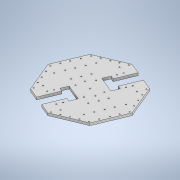
# Autodesk Inventor part: Support bas
Saved by Autodesk Inventor 2020 (Build 240168000, 168)
## iProperties
Created: 2019-11-28
Part Number: Support bas
Material: Générique
Document SubType Name: Modeling
Designer: erwan
Density: 1 g/cm^3
Appearance: Par défaut
Author: erwan
Autodesk Inventor part; units mm, degrees
ref_plane "YZ Plane" through (0, 0, 0) normal (1, 0, 0) x (0, 1, 0)
ref_plane "XZ Plane" through (0, 0, 0) normal (0, 1, 0) x (-1, 0, 0)
ref_plane "XY Plane" through (0, 0, 0) normal (0, 0, 1) x (1, 0, 0)
sketch "Esquisse1" plane through (0, 0, 0) normal (0, 1, 0) x (-1, 0, 0)
  line L0 (174.5381, 0.1913) -> (123.2817, 123.935)
  line L1 (174.5381, 0.1913) -> (123.2817, -123.5523)
  line L2 (123.2817, -123.5523) -> (-0.4619, -174.8087)
  line L3 (-123.2817, -123.935) -> (-174.5381, -0.1913)
  line L4 (-174.5381, -0.1913) -> (-123.2817, 123.5523)
  line L5 (-123.2817, 123.5523) -> (0.4619, 174.8087)
  line L6 (-0.4619, -174.8087) -> (-43.3943, -157.0255)
  line L7 (-123.2817, -123.935) -> (-80.3494, -141.7182)
  line L8 (-1.0786, 88.8554) -> (-12.5591, 61.139)
  line L9 (-12.5591, 61.139) -> (52.1124, 34.3512)
  line L10 (52.1124, 34.3512) -> (63.593, 62.0676)
  line L11 (63.593, 62.0676) -> (49.7348, 67.8078)
  line L12 (49.7348, 67.8078) -> (80.3494, 141.7182)
  line L13 (-1.0786, 88.8554) -> (12.7796, 83.1151)
  line L14 (12.7796, 83.1151) -> (43.3943, 157.0255)
  line L15 (123.2817, 123.935) -> (80.3494, 141.7182)
  line L16 (0.4619, 174.8087) -> (43.3943, 157.0255)
  line L17 (-63.593, -62.0676) -> (-52.1124, -34.3512)
  line L18 (-52.1124, -34.3512) -> (12.5591, -61.139)
  line L19 (12.5591, -61.139) -> (1.0786, -88.8554)
  line L20 (1.0786, -88.8554) -> (-12.7796, -83.1151)
  line L21 (-12.7796, -83.1151) -> (-43.3943, -157.0255)
  line L22 (-63.593, -62.0676) -> (-49.7348, -67.8078)
  line L23 (-49.7348, -67.8078) -> (-80.3494, -141.7182)
  point P0 (0, 0)
  dimension "d113" = 30
  dimension "d114" = 70
  dimension "d115" = 30
  dimension "d116" = 15
  dimension "d117" = 15
  dimension "d120" = 30
  dimension "d121" = 70
  dimension "d122" = 15
  dimension "d123" = 15
  constraints: 48 end point, 8 perpendicular, 2 collinear
  measures "d113" distance of L8.start L8.end
  measures "d114" distance of L8.end L9.end
  measures "d115" distance of L9.end L10.end
  measures "d116" distance of L10.end L11.end
  measures "d117" distance of L8.start L13.end
  measures "d120" distance of L17.start L17.end
  measures "d121" distance of L17.end L18.end
  measures "d122" distance of L19.end L20.end
  measures "d123" distance of L17.start L22.end
extrude "Extrusion1" add sketch "Esquisse1" along normal blind 10
sketch "Esquisse2" plane through (0, 10, 0) normal (0, 1, 0) x (1, 0, 0)
  line L0 (0, 0) -> (135.5137, -56.1316) construction
  line L1 (0, 0) -> (-162.1857, 67.1795) construction
  line L2 (0, 175) -> (-123.7437, -123.7437) construction
  line L3 (0, -175) -> (123.7437, 123.7437) construction
  line L4 (174.5381, 0.1913) -> (-123.2817, 123.5523) construction
  line L5 (-174.5381, -0.1913) -> (123.2817, -123.5523) construction
  line L6 (150.0138, 60.7587) -> (-149.0913, -62.1087) construction
  line L7 (-60.9725, 148.8775) -> (61.8949, -150.2276) construction
  line L8 (-60.9725, 148.8775) -> (-149.0913, -62.1087) construction
  line L9 (61.8949, -150.2276) -> (150.0138, 60.7587) construction
  circle A0 centre (165.8145, -1.0193) radius 2.25
  line L10 (165.8145, -1.0193) -> (116.2638, -120.6454) construction
  circle A1 centre (116.2638, -120.6454) radius 2.25
  circle A2 centre (141.8919, -58.7736) radius 2.25
  circle A3 centre (153.2932, -30.2913) radius 2.25
  circle A4 centre (128.2212, -90.3222) radius 2.25
  line L11 (119.9169, 114.5049) -> (165.8145, -1.0193) construction
  circle A5 centre (119.9169, 114.5049) radius 2.25
  circle A6 centre (142.4969, 57.6709) radius 2.25
  circle A7 centre (130.8905, 86.6335) radius 2.25
  circle A8 centre (153.432, 29.381) radius 2.25
  line L12 (3.8268, -165.7612) -> (116.2638, -120.6454) construction
  circle A9 centre (3.8268, -165.7612) radius 2.25
  circle A10 centre (60.0453, -143.2033) radius 2.25
  circle A11 centre (31.6722, -154.3729) radius 2.25
  circle A12 centre (87.3628, -131.5964) radius 2.25
  line L13 (-164.5381, -0.1913) -> (-114.7462, 120.0168) construction
  circle A13 centre (-164.5381, -0.1913) radius 2.25
  circle A14 centre (-114.7462, 120.0168) radius 2.25
  circle A15 centre (-140.3744, 58.145) radius 2.25
  circle A16 centre (-127.2988, 88.9721) radius 2.25
  circle A17 centre (-152.3708, 28.9413) radius 2.25
  line L14 (-3.8268, 165.7612) -> (-114.7462, 120.0168) construction
  circle A18 centre (-3.8268, 165.7612) radius 2.25
  circle A19 centre (-58.6246, 143.162) radius 2.25
  circle A20 centre (-31.6722, 154.3729) radius 2.25
  circle A21 centre (-87.3628, 131.5964) radius 2.25
  line L15 (-119.9169, -114.5049) -> (-164.5381, -0.1913) construction
  circle A22 centre (-119.9169, -114.5049) radius 2.25
  circle A23 centre (-141.5745, -59.0209) radius 2.25
  circle A24 centre (-130.8905, -86.6335) radius 2.25
  circle A25 centre (-153.432, -29.381) radius 2.25
  circle A26 centre (15.3073, -138.0448) radius 2.25
  circle A27 centre (80.4463, -105.8093) radius 2.25
  circle A28 centre (105.9544, -44.7345) radius 2.25
  circle A29 centre (132.0654, 17.7841) radius 2.25
  circle A30 centre (108.4363, 86.7885) radius 2.25
  circle A31 centre (61.8718, -25.6282) radius 2.25
  circle A32 centre (0, 0) radius 2.25
  circle A33 centre (-15.3073, 138.0448) radius 2.25
  circle A34 centre (-79.1792, 105.2845) radius 2.25
  circle A35 centre (-105.0319, 43.3844) radius 2.25
  circle A36 centre (-130.7983, -18.309) radius 2.25
  circle A37 centre (-61.8718, 25.6282) radius 2.25
  line L16 (183.0548, 10.7676) -> (-121.8254, 137.0531) construction
  line L17 (-121.8254, 137.0531) -> (-183.0548, -10.7676) construction
  line L18 (-183.0548, -10.7676) -> (121.8254, -137.0531) construction
  line L19 (183.0548, 10.7676) -> (121.8254, -137.0531) construction
  line L20 (15.3073, -138.0448) -> (-145.3915, -71.4812) construction
  line L21 (15.3073, -138.0448) -> (52.2625, -153.3522) construction
  circle A38 centre (-108.4363, -86.7885) radius 2.25
  line L22 (-15.6478, 66.748) -> (-57.8915, -35.2375) construction
  line L23 (58.2626, 36.1333) -> (15.8255, -66.3188) construction
  circle A39 centre (37.0441, -15.0928) radius 2.25
  circle A40 centre (-36.7697, 15.7552) radius 2.25
  line L24 (31.2572, -99.5385) -> (49.7348, -107.1922) construction
  line L25 (49.7348, -107.1922) -> (42.0811, -125.6698) construction
  line L26 (42.0811, -125.6698) -> (23.6035, -118.0161) construction
  line L27 (31.2572, -99.5385) -> (23.6035, -118.0161) construction
  line L28 (92.4865, 48.2822) -> (110.9641, 40.6285) construction
  line L29 (110.9641, 40.6285) -> (118.6178, 59.1061) construction
  line L30 (118.6178, 59.1061) -> (100.1402, 66.7598) construction
  line L31 (92.4865, 48.2822) -> (100.1402, 66.7598) construction
  line L32 (-92.4865, -48.2822) -> (-110.9641, -40.6285) construction
  line L33 (-110.9641, -40.6285) -> (-118.6178, -59.1061) construction
  line L34 (-118.6178, -59.1061) -> (-100.1402, -66.7598) construction
  line L35 (-92.4865, -48.2822) -> (-100.1402, -66.7598) construction
  line L36 (-31.2572, 99.5385) -> (-23.6035, 118.0161) construction
  line L37 (-23.6035, 118.0161) -> (-42.0811, 125.6698) construction
  line L38 (-42.0811, 125.6698) -> (-49.7348, 107.1922) construction
  line L39 (-31.2572, 99.5385) -> (-49.7348, 107.1922) construction
  line L40 (-152.3708, 28.9413) -> (128.2212, -90.3222) construction
  line L41 (153.2932, -30.2913) -> (-127.2988, 88.9721) construction
  circle A41 centre (-117.2914, 14.0311) radius 2.25
  circle A42 centre (-92.2194, 74.0619) radius 2.25
  circle A43 centre (118.2139, -15.3811) radius 2.25
  circle A44 centre (93.1419, -75.412) radius 2.25
  circle A45 centre (49.0189, -56.6578) radius 2.25
  circle A46 centre (-74.2528, -4.2622) radius 2.25
  circle A47 centre (-49.3563, 55.8433) radius 2.25
  circle A48 centre (73.9154, 3.4476) radius 2.25
  circle A49 centre (-41.8248, -18.0454) radius 2.25
  circle A50 centre (-17.1286, 42.1451) radius 2.25
  circle A51 centre (42.7473, 16.6954) radius 2.25
  circle A52 centre (18.051, -43.4952) radius 2.25
  line L42 (12.5591, -61.139) -> (1.0786, -88.8554) projected
  line L43 (1.0786, -88.8554) -> (-29.4222, -162.8129) construction
  line L44 (-43.3943, -157.0255) -> (-0.4619, -174.8087) projected
  line L45 (-63.593, -62.0676) -> (-52.1124, -34.3512) projected
  line L46 (-63.593, -62.0676) -> (-94.4694, -135.8695) construction
  line L47 (-123.2817, -123.935) -> (-80.3494, -141.7182) projected
  line L48 (-100.1402, -66.7598) -> (23.6035, -118.0161) construction
  line L49 (-12.7796, -83.1151) -> (-43.3943, -157.0255) projected
  line L50 (-23.6035, 118.0161) -> (100.1402, 66.7598) construction
  line L51 (-1.0786, 88.8554) -> (29.7527, 162.676) construction
  line L52 (63.2824, 61.9749) -> (93.8612, 136.1214) construction
  line L53 (123.2817, 123.935) -> (80.3494, 141.7182) projected
  line L54 (-15.3073, 138.0448) -> (108.4363, 86.7885) construction
  circle A53 centre (-79.0312, -98.9685) radius 2.25
  circle A54 centre (-70.6641, -78.9692) radius 2.25
  circle A55 centre (-5.9065, -105.7927) radius 2.25
  circle A56 centre (-14.1718, -125.8342) radius 2.25
  circle A57 centre (14.3371, 125.7657) radius 2.25
  circle A58 centre (5.9822, 105.7613) radius 2.25
  circle A59 centre (70.3455, 79.1012) radius 2.25
  circle A60 centre (78.6108, 99.1427) radius 2.25
  dimension "d14" = 4.5
  dimension "d15" = 4.5
  dimension "d16" = 4.5
  dimension "d17" = 4.5
  dimension "d18" = 4.5
  dimension "d19" = 10
  dimension "d20" = 4.5
  dimension "d21" = 4.5
  dimension "d22" = 4.5
  dimension "d23" = 4.5
  dimension "d24" = 10
  dimension "d25" = 4.5
  dimension "d26" = 4.5
  dimension "d27" = 4.5
  dimension "d28" = 4.5
  dimension "d29" = 10
  dimension "d30" = 4.5
  dimension "d31" = 4.5
  dimension "d32" = 4.5
  dimension "d33" = 4.5
  dimension "d34" = 4.5
  dimension "d35" = 10
  dimension "d36" = 4.5
  dimension "d37" = 4.5
  dimension "d38" = 4.5
  dimension "d39" = 4.5
  dimension "d40" = 10
  dimension "d41" = 4.5
  dimension "d42" = 4.5
  dimension "d43" = 4.5
  dimension "d44" = 4.5
  dimension "d45" = 4.5
  dimension "d46" = 4.5
  dimension "d47" = 4.5
  dimension "d48" = 4.5
  dimension "d49" = 4.5
  dimension "d51" = 4.5
  dimension "d53" = 4.5
  dimension "d54" = 4.5
  dimension "d56" = 4.5
  dimension "d57" = 4.5
  dimension "d58" = 4.5
  dimension "d60" = 4.5
  dimension "d68" = 330
  dimension "d69" = 160
  dimension "d82" = 4.5
  dimension "d85" = 4.5
  dimension "d86" = 4.5
  dimension "d87" = 20
  dimension "d88" = 20
  dimension "d89" = 20
  dimension "d90" = 20
  dimension "d91" = 20
  dimension "d92" = 20
  dimension "d93" = 20
  dimension "d94" = 20
  dimension "d95" = 4.5
  dimension "d96" = 4.5
  dimension "d97" = 4.5
  dimension "d98" = 4.5
  dimension "d99" = 4.5
  dimension "d100" = 4.5
  dimension "d101" = 4.5
  dimension "d102" = 4.5
  constraints: 94 end point, 66 point on line, 61 centre point, 10 perpendicular, 8 coincident, 8 midpoint, 1 collinear, 1 parallel, 32 other
  measures "d14" diameter of A0
  measures "d15" diameter of A1
  measures "d16" diameter of A2
  measures "d17" diameter of A3
  measures "d18" diameter of A4
  measures "d19" distance of point (123.744, 123.744) L11.start
  measures "d20" diameter of A5
  measures "d21" diameter of A6
  measures "d22" diameter of A7
  measures "d23" diameter of A8
  measures "d24" distance of point (0, -175) L12.start
  measures "d25" diameter of A9
  measures "d26" diameter of A10
  measures "d27" diameter of A11
  measures "d28" diameter of A12
  measures "d29" distance of L5.start L13.start
  measures "d30" diameter of A13
  measures "d31" diameter of A14
  measures "d32" diameter of A15
  measures "d33" diameter of A16
  measures "d34" diameter of A17
  measures "d35" distance of point (0, 175) L14.start
  measures "d36" diameter of A18
  measures "d37" diameter of A19
  measures "d38" diameter of A20
  measures "d39" diameter of A21
  measures "d40" distance of point (-123.744, -123.744) L15.start
  measures "d41" diameter of A22
  measures "d42" diameter of A23
  measures "d43" diameter of A24
  measures "d44" diameter of A25
  measures "d45" diameter of A26
  measures "d46" diameter of A27
  measures "d47" diameter of A28
  measures "d48" diameter of A29
  measures "d49" diameter of A30
  measures "d51" diameter of A31
  measures "d53" diameter of A32
  measures "d54" diameter of A33
  measures "d56" diameter of A34
  measures "d57" diameter of A35
  measures "d58" diameter of A36
  measures "d60" diameter of A37
  measures "d68" distance of L16.start L16.end
  measures "d69" distance of L16.end L17.end
  measures "d82" diameter of A38
  measures "d85" diameter of A39
  measures "d86" diameter of A40
  measures "d87" distance of L24.start L24.end
  measures "d88" distance of L24.end L25.end
  measures "d89" distance of L28.start L28.end
  measures "d90" distance of L28.end L29.end
  measures "d91" distance of L32.start L32.end
  measures "d92" distance of L32.end L33.end
  measures "d93" distance of L36.start L36.end
  measures "d94" distance of L36.end L37.end
  measures "d95" diameter of A41
  measures "d96" diameter of A42
  measures "d97" diameter of A43
  measures "d98" diameter of A44
  measures "d99" diameter of A45
  measures "d100" diameter of A46
  measures "d101" diameter of A47
  measures "d102" diameter of A48
extrude "Extrusion2" cut sketch "Esquisse2" against normal blind 10
